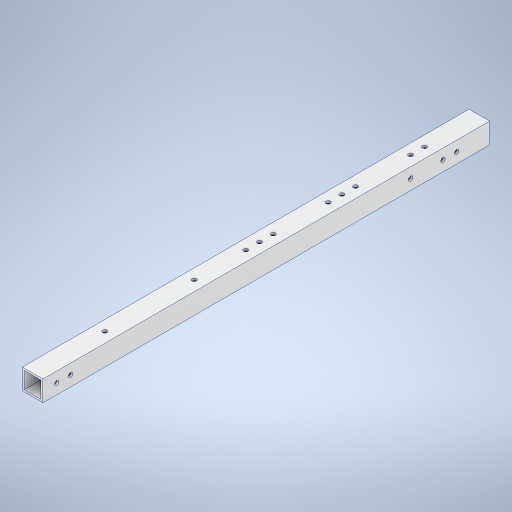
# Autodesk Inventor part: 射出_角柱2
Saved by Autodesk Inventor 2023 (Build 270158000, 158)
## iProperties
Created: 2022-04-20
Part Number: 射出_角柱2
Material: アルミニウム 6061
Document SubType Name: Modeling
Designer: yuta
Density: 2.7 g/cm^3
Appearance: アルミニウム - フラット
Author: yuta
Autodesk Inventor part; units mm, degrees
ref_plane "YZ Plane" through (0, 0, 0) normal (1, 0, 0) x (0, 1, 0)
ref_plane "XZ Plane" through (0, 0, 0) normal (0, 1, 0) x (-1, 0, 0)
ref_plane "XY Plane" through (0, 0, 0) normal (0, 0, 1) x (1, 0, 0)
sketch "スケッチ1" plane through (0, 0, 0) normal (0, 0, 1) x (1, 0, 0)
  line L0 (0, 0) -> (15, 0)
  line L1 (15, 0) -> (15, 15)
  line L2 (15, 15) -> (0, 15)
  line L3 (0, 15) -> (0, 0)
  dimension "d0" = 15
  dimension "d1" = 15
  constraints: 8 end point, 2 parallel, 1 horizontal, 1 perpendicular
  measures "d0" distance of L2.end L1.end
  measures "d1" distance of L1.end L0.end
extrude "押し出し1" add sketch "スケッチ1" along normal blind 140
sketch "スケッチ2" plane through (0, 15, 0) normal (0, 1, 0) x (1, 0, 0)
  line L0 (0, 0) -> (0, -140) construction
  line L1 (15, -80) -> (15, -65) construction
  line L2 (15, -65) -> (0, -65) construction
  circle A0 centre (7.5, -72.5) radius 1.6
  line L3 (15, 0) -> (15, -140) construction
  line L4 (15, 0) -> (0, 0) construction
  line L5 (0, 0) -> (0, -15) construction
  line L6 (0, -15) -> (15, -15) construction
  line L7 (15, -15) -> (15, 0) construction
  circle A1 centre (7.5, -7.5) radius 1.6
  dimension "d5" = 15
  dimension "d6" = 15
  dimension "d7" = 3.2
  dimension "d8" = 15
  dimension "d9" = 15
  dimension "d10" = 3.2
  constraints: 12 end point, 2 centre point, 2 horizontal, 2 parallel, 2 vertical, 1 perpendicular, 4 other
  measures "d5" distance of L2.end L1.end
  measures "d6" distance of L1.end L1.start
  measures "d7" diameter of A0
  measures "d8" distance of L6.end L5.end
  measures "d9" distance of L5.end L4.end
  measures "d10" diameter of A1
hole "穴1" at (7.5, 15, 72.5) at (7.5, 15, 7.5) direction (0, -1, 0) diameter 3.2 end through all
sketch "スケッチ3" plane through (0, 0, 0) normal (0, 0, -1) x (-1, 0, 0)
  line L0 (0, 0) -> (-15, 0)
  line L1 (-15, 0) -> (-15, 15)
  line L2 (-15, 15) -> (0, 15)
  line L3 (0, 15) -> (0, 0)
  dimension "d18" = 15
  dimension "d19" = 15
  constraints: 8 end point, 2 parallel, 1 horizontal, 1 perpendicular
  measures "d18" distance of L1.end L2.end
  measures "d19" distance of L0.end L1.end
extrude "押し出し2" add sketch "スケッチ3" along normal blind 200
sketch "スケッチ4" plane through (0, 0, -200) normal (0, 0, -1) x (-1, 0, 0)
  point P0 (0, 0)
sketch "スケッチ5" plane through (0, 0, -200) normal (0, 0, -1) x (-1, 0, 0)
  line L0 (0, 0) -> (-15, 0) projected
  line L1 (0, 0) -> (-15, 0)
  line L2 (-15, 0) -> (-15, 15)
  line L3 (-15, 15) -> (0, 15)
  line L4 (0, 15) -> (0, 0)
  dimension "d22" = 15
  dimension "d23" = 15
  constraints: 8 end point, 2 parallel, 1 horizontal, 1 perpendicular
  measures "d22" distance of L2.end L3.end
  measures "d23" distance of L1.end L2.end
extrude "押し出し3" cut sketch "スケッチ5" against normal blind 15
sketch "スケッチ6" plane through (0, 0, -185) normal (0, 0, -1) x (-1, 0, 0)
  line L0 (0, 15) -> (0, 0) projected
  line L1 (0, 0) -> (-15, 0)
  line L2 (-15, 0) -> (-15, 15)
  line L3 (-15, 15) -> (0, 15)
  line L4 (0, 15) -> (0, 0)
  dimension "d26" = 15
  dimension "d27" = 15
  constraints: 8 end point, 2 parallel, 1 horizontal, 1 perpendicular
  measures "d26" distance of L2.end L3.end
  measures "d27" distance of L1.end L2.end
extrude "押し出し4" add sketch "スケッチ6" along normal blind 15
sketch "スケッチ7" plane through (0, 0, 140) normal (0, 0, 1) x (1, 0, 0)
  line L0 (0, 0) -> (15, 0)
  line L1 (15, 0) -> (15, 15)
  line L2 (15, 15) -> (0, 15)
  line L3 (0, 15) -> (0, 0)
  dimension "d30" = 15
  dimension "d31" = 15
  constraints: 8 end point, 2 parallel, 1 horizontal, 1 perpendicular
  measures "d30" distance of L2.end L1.end
  measures "d31" distance of L1.end L0.end
extrude "押し出し5" cut sketch "スケッチ7" against normal blind 15
sketch "スケッチ9" plane through (15, 0, -200) normal (1, 0, 0) x (0, 0, -1)
  circle A0 centre (-315, 7.5) radius 1.6
  line L0 (-325, 15) -> (-325, 0) projected
  line L1 (-325, 0) -> (0, 0) projected
  point P0 (-200, 0)
  dimension "d44" = 3.2
  dimension "d45" = 10
  dimension "d46" = 7.5
  constraints: 1 centre point
  measures "d44" diameter of A0
  measures "d45" distance from line of L0 A0.centre
  measures "d46" distance from line of L1 A0.centre
hole "穴3" at (15, 7.5, 115) direction (-1, 0, 0) diameter 3.2 end through all
sketch "スケッチ10" plane through (15, 0, -200) normal (1, 0, 0) x (0, 0, -1)
  circle A0 centre (-315, 7.5) radius 1.6 projected
  line L0 (-325, 0) -> (0, 0) projected
  point P0 (-200, 0)
  point P1 (-305, 7.5)
  dimension "d54" = 10
  dimension "d55" = 7.5
  measures "d54" distance of A0.centre point (-305, 7.5)
  measures "d55" distance from line of L0 point (-305, 7.5)
hole "穴4" at (15, 7.5, 105) direction (-1, 0, 0) diameter 3.2 end through all
sketch "スケッチ11" plane through (15, 0, -200) normal (1, 0, 0) x (0, 0, -1)
  line L0 (0, 15) -> (0, 0) projected
  line L1 (0, 15) -> (-325, 15) projected
  point P0 (-200, 0)
  point P1 (-24, 7.5)
  point P2 (-34, 7.5)
  dimension "d63" = 24
  dimension "d64" = 7.5
  dimension "d65" = 10
  dimension "d66" = 7.5
  measures "d63" distance from line of L0 point (-24, 7.5)
  measures "d64" distance from line of L1 point (-24, 7.5)
  measures "d65" distance of point (-34, 7.5) point (-24, 7.5)
  measures "d66" distance from line of L1 point (-34, 7.5)
hole "穴5" at (15, 7.5, -166) at (15, 7.5, -176) direction (-1, 0, 0) diameter 3.2 end through all
sketch "スケッチ12" plane through (0, 15, -200) normal (0, 1, 0) x (1, 0, 0)
  line L0 (0, 0) -> (15, 0) projected
  point P0 (0, -200)
  point P1 (7.5, -40)
  point P2 (7.5, -50)
  point P3 (7.5, -90)
  point P4 (7.5, -100)
  point P5 (7.5, -110)
  point P6 (7.5, -150)
  point P7 (7.5, -160)
  point P8 (7.5, -170)
  dimension "d74" = 40
  dimension "d75" = 7.5
  dimension "d76" = 10
  dimension "d77" = 90
  dimension "d78" = 10
  dimension "d79" = 10
  dimension "d80" = 150
  dimension "d81" = 10
  dimension "d82" = 10
  measures "d74" distance from line of L0 point (7.5, -40)
  measures "d75" horizontal distance of L0.end point (7.5, -40)
  measures "d76" distance of point (7.5, -40) point (7.5, -50)
  measures "d77" distance from line of L0 point (7.5, -90)
  measures "d78" distance of point (7.5, -90) point (7.5, -100)
  measures "d79" distance of point (7.5, -100) point (7.5, -110)
  measures "d80" distance from line of L0 point (7.5, -150)
  measures "d81" distance of point (7.5, -150) point (7.5, -160)
  measures "d82" distance of point (7.5, -160) point (7.5, -170)
hole "穴6" at (7.5, 15, -30) at (7.5, 15, -40) at (7.5, 15, -50) at (7.5, 15, -90) at (7.5, 15, -100) at (7.5, 15, -110) at (7.5, 15, -150) at (7.5, 15, -160) direction (0, -1, 0) diameter 3.2 end through all
sketch "スケッチ13" plane through (0, 0, 125) normal (0, 0, 1) x (1, 0, 0)
  line L0 (1.5, 13.5) -> (13.5, 13.5)
  line L1 (13.5, 13.5) -> (13.5, 1.5)
  line L2 (13.5, 1.5) -> (1.5, 1.5)
  line L3 (1.5, 1.5) -> (1.5, 13.5)
  line L4 (0, 0) -> (0, 15) projected
  line L5 (0, 15) -> (15, 15) projected
  dimension "d90" = 12
  dimension "d91" = 12
  dimension "d92" = 1.5
  dimension "d93" = 1.5
  constraints: 8 end point, 2 parallel, 1 horizontal, 1 perpendicular
  measures "d90" distance of L1.end L2.end
  measures "d91" distance of L0.end L1.end
  measures "d92" distance between parallel lines of L4 L3
  measures "d93" distance between parallel lines of L5 L0
extrude "押し出し6" cut sketch "スケッチ13" against normal blind 340
sketch "スケッチ14" plane through (15, 0, -200) normal (1, 0, 0) x (0, 0, -1)
  line L0 (0, 15) -> (0, 0) projected
  line L1 (0, 15) -> (-325, 15) projected
  point P0 (-200, 0)
  point P1 (-57.5, 7.5)
  dimension "d96" = 57.5
  dimension "d97" = 7.5
  measures "d96" distance from line of L0 point (-57.5, 7.5)
  measures "d97" distance from line of L1 point (-57.5, 7.5)
hole "穴7" at (15, 7.5, -142.5) direction (-1, 0, 0) diameter 3.2 end through all
